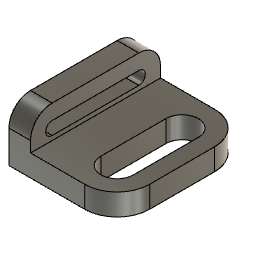
Model 7 (Autodesk Fusion 360 design; units mm, degrees)
Autodesk Fusion 360 part; units mm, degrees
sketch "Sketch5" plane through (0, 0, 0) normal (0, 0, 1) x (1, 0, 0)
  line L0 (0, 0) -> (70, 0)
  line L1 (70, 0) -> (70, 120) construction
  line L2 (70, 120) -> (0, 120)
  line L3 (0, 120) -> (0, 0)
  line L4 (0, 120) -> (20, 120) construction
  line L5 (20, 120) -> (20, 0)
  line L6 (70, 120) -> (70, 90) construction
  line L7 (70, 0) -> (70, 30) construction
  line L8 (100, 90) -> (100, 30)
  line L9 (85, 90) -> (85, 30)
  line L10 (55, 90) -> (55, 30)
  arc A0 (100, 90) -> (70, 120) centre (70, 90) ccw
  arc A1 (70, 0) -> (100, 30) centre (70, 30) ccw
  arc A2 (85, 90) -> (55, 90) centre (70, 90) ccw
  arc A3 (55, 30) -> (85, 30) centre (70, 30) ccw
  dimension "d21" = 70
  dimension "d22" = 120
  dimension "d23" = 20
  dimension "d24" = 30
  dimension "d25" = 30
  dimension "d26" = 30
  dimension "d27" = 60
  dimension "d28" = 30
  dimension "d29" = 60
  constraint horizontal L0
  constraint vertical L1
  constraint horizontal L2
  constraint vertical L3
  constraint coincident L0.start L3.end
  constraint perpendicular L3 L4
  constraint coincident L0 L5.end
  constraint perpendicular L0 L5
  constraint coincident L1 L6.end
  constraint perpendicular L0 L7
  constraint coincident L6.end A0.centre
  constraint concentric A0 A2
  constraint coincident L7.end A1.centre
  constraint concentric A1 A3
  constraint tangent L8 A1
  constraint vertical L8
  constraint tangent L9 A3
  constraint parallel L8 L9
  constraint tangent L10 A3
  constraint parallel L9 L10
  measures "d21" distance of L0.start L0.end
  measures "d22" distance of L0.start L2.end
  measures "d23" distance of L2.end L4.end
  measures "d24" distance of L1.end L6.end
  measures "d25" distance of L0.end L7.end
  measures "d26" diameter of A2
  measures "d27" diameter of A0
  measures "d28" diameter of A3
  measures "d29" diameter of A1
extrude "Extrude3" add sketch "Sketch5" along normal blind 20 contours L0 L2 L5 L8 A0 A1
ref_plane "WorkPlane1" through (20, 0, 0) normal (1, 0, 0) x (0, 1, 0)
sketch "Sketch6" plane through (20, 0, 0) normal (1, 0, 0) x (0, 1, 0)
  line L0 (0, 30) -> (0, 50) construction
  line L1 (0, 30) -> (20, 30) construction
  line L2 (20, 30) -> (20, 36) construction
  line L3 (20, 36) -> (96.6834, 36)
  line L4 (100, 24) -> (20, 24)
  arc A0 (20, 36) -> (20, 24) centre (20, 30) ccw
  line L5 (20, 30) -> (20, 50) construction
  line L6 (20, 50) -> (100, 50)
  arc A1 (20, 50) -> (0, 30) centre (20, 30) ccw
  line L7 (120, 0) -> (120, 30)
  line L8 (120, 30) -> (120, 50) construction
  line L9 (120, 30) -> (100, 30) construction
  line L10 (96.6834, 36) -> (100, 36)
  arc A2 (120, 30) -> (100, 50) centre (100, 30) ccw
  line L11 (0, 30) -> (0, 0)
  arc A3 (100, 24) -> (100, 36) centre (100, 30) ccw
  line L12 (120, 0) -> (0, 0)
  dimension "d33" = 20
  dimension "d34" = 30
  dimension "d35" = 20
  dimension "d36" = 12
  dimension "d37" = 40
  dimension "d44" = 30
  dimension "d45" = 20
  dimension "d46" = 20
  dimension "d47" = 12
  dimension "d48" = 40
  dimension "d49" = 80
  constraint coincident L1.end L2.start
  constraint perpendicular L1 L2
  constraint perpendicular L2 L3
  constraint tangent L4 A0
  constraint perpendicular L1 L5
  constraint vertical L7
  constraint parallel L7 L8
  constraint coincident L9.end A2.centre
  constraint tangent L10 A3
  constraint parallel L3 L10
  constraint coincident L11.end L12.end
  constraint perpendicular L1 L11
  constraint perpendicular L11 L12
  measures "d33" distance of L0.start L0.end
  measures "d34" distance of L11.end L0.start
  measures "d35" distance of L0.start L1.end
  measures "d36" diameter of A0
  measures "d37" diameter of A1
  measures "d44" distance of L7.start L7.end
  measures "d45" distance of L7.end L8.end
  measures "d46" distance of L7.end L9.end
  measures "d47" diameter of A3
  measures "d48" diameter of A2
  measures "d49" distance of L1.end L9.end
extrude "Extrude4" add sketch "Sketch6" against normal blind 20
